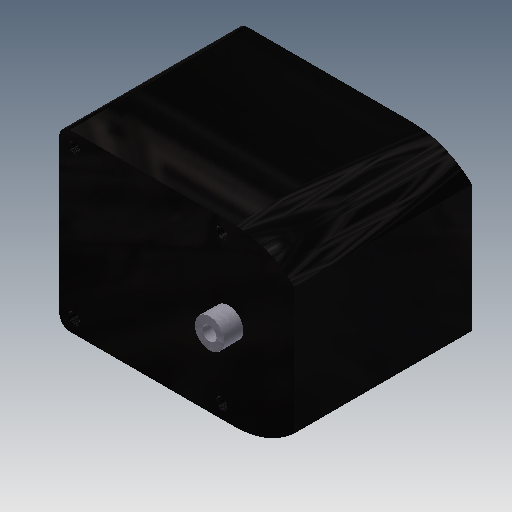
# Autodesk Inventor part: KRS-4034HV
Saved by Autodesk Inventor 2019.4 (Build 234330000, 330)
## iProperties
Created: 2017-04-05
Part Number: KRS-4034HV
Material: アセタール樹脂、黒
Document SubType Name: Modeling
Designer: Owner
Density: 1.41547 g/cm^3
Appearance: 滑らか - 黒
Mass: 61.2 g
Surface Area: 86.4058 cm^2
Volume: 43.2365 cm^3
Author: Owner
Autodesk Inventor part; units mm, degrees
ref_plane "YZ Plane" through (0, 0, 0) normal (1, 0, 0) x (0, 1, 0)
ref_plane "XZ Plane" through (0, 0, 0) normal (0, 1, 0) x (-1, 0, 0)
ref_plane "XY Plane" through (0, 0, 0) normal (0, 0, 1) x (1, 0, 0)
sketch "スケッチ1" plane through (0, 0, 0) normal (0, 0, 1) x (1, 0, 0)
  line L0 (-37.5496, 23.6801) -> (-7.5496, 23.6801)
  line L1 (3.4504, 19.2991) -> (3.4504, -3.9388)
  line L2 (-7.5496, -8.3199) -> (-37.5496, -8.3199)
  line L3 (-39.5496, -6.3199) -> (-39.5496, 21.6801)
  circle A0 centre (-36.8093, -5.8199) radius 1.05
  circle A1 centre (-36.8093, 21.1801) radius 1.05
  arc A2 (-37.5496, 23.6801) -> (-39.5496, 21.6801) centre (-37.5496, 21.6801) ccw
  arc A3 (-39.5496, -6.3199) -> (-37.5496, -8.3199) centre (-37.5496, -6.3199) ccw
  circle A4 centre (-9.8093, -5.8199) radius 1.05
  circle A5 centre (-9.8093, 21.1801) radius 1.05
  line L4 (-39.5496, 7.6801) -> (3.4504, 7.6801) construction
  line L5 (-17.0496, 23.6801) -> (-17.0496, -8.3199) construction
  arc A6 (-7.5496, -8.3199) -> (3.4504, -3.9388) centre (-7.5496, 7.6801) ccw
  arc A7 (3.4504, 19.2991) -> (-7.5496, 23.6801) centre (-7.5496, 7.6801) ccw
  point P0 (-39.5496, -8.3199)
  point P1 (-17.0496, 7.6801)
  dimension "d23" = 2.1
  dimension "d24" = 2.1
  dimension "d25" = 27
  dimension "d26" = 2.5
  dimension "d27" = 2.5
  dimension "d28" = 2
  dimension "d31" = 2.1
  dimension "d32" = 2.1
  dimension "d33" = 27
  dimension "d34" = 27
  constraints: 12 end point, 8 centre point, 8 point on circle, 4 point on line, 4 tangent, 3 midpoint, 2 parallel, 1 equal radius, 1 horizontal, 1 perpendicular
  measures "d23" diameter of A0
  measures "d24" diameter of A1
  measures "d25" distance of A0.centre A1.centre
  measures "d26" distance from line of L0 A1.centre
  measures "d27" distance from line of L2 A0.centre
  measures "d28" radius of A2
  measures "d31" diameter of A4
  measures "d32" diameter of A5
  measures "d33" distance of A0.centre A4.centre
  measures "d34" distance of A5.centre A1.centre
extrude "押し出し1" add sketch "スケッチ1" along normal blind 32.5
sketch "スケッチ2" plane through (0, 0, 32.5) normal (0, 0, 1) x (1, 0, 0)
  circle A0 centre (-9.8093, 21.1801) radius 1.05 projected
  circle A1 centre (-9.8093, -5.8199) radius 1.05 projected
  circle A2 centre (-36.8093, 21.1801) radius 1.05 projected
  circle A3 centre (-36.8093, -5.8199) radius 1.05 projected
  line L0 (3.4504, -3.9388) -> (3.4504, 19.2991) projected
  arc A4 (3.4504, 19.2991) -> (-7.5496, 23.6801) centre (-7.5496, 7.6801) ccw projected
  line L1 (-7.5496, 23.6801) -> (-37.5496, 23.6801) projected
  arc A5 (-37.5496, 23.6801) -> (-39.5496, 21.6801) centre (-37.5496, 21.6801) ccw projected
  line L2 (-39.5496, 21.6801) -> (-39.5496, -6.3199) projected
  arc A6 (-39.5496, -6.3199) -> (-37.5496, -8.3199) centre (-37.5496, -6.3199) ccw projected
  line L3 (-37.5496, -8.3199) -> (-7.5496, -8.3199) projected
  arc A7 (-7.5496, -8.3199) -> (3.4504, -3.9388) centre (-7.5496, 7.6801) ccw projected
  line L4 (-39.5496, 21.6801) -> (-39.5496, -6.3199) construction
  line L5 (-39.5496, 7.6801) -> (3.4504, 7.6801) construction
  line L6 (-7.5496, -8.3199) -> (-37.5496, -8.3199) construction
  line L7 (-18.0496, -8.3199) -> (-18.0496, 23.6801) construction
  line L8 (-7.5496, 23.6801) -> (-37.5496, 23.6801) construction
  circle A8 centre (-8.55, 7.6801) radius 2.7
  circle A9 centre (-8.55, 7.6801) radius 1.3
  point P0 (0, 0)
  dimension "d49" = 5.4
  dimension "d50" = 2.6
  dimension "d51" = 9.4996
  constraints: 4 end point, 3 point on line, 2 centre point, 2 coincident, 2 midpoint, 1 perpendicular
  measures "d49" diameter of A8
  measures "d50" diameter of A9
  measures "d51" distance from line of L7 A8.centre
extrude "押し出し3" add sketch "スケッチ2" along normal blind 3.5 contours A8
sketch "スケッチ3" plane through (0, 0, 0) normal (0, 0, -1) x (-1, 0, 0)
  circle A0 centre (9.8093, 21.1801) radius 1.05 projected
  circle A1 centre (9.8093, -5.8199) radius 1.05 projected
  circle A2 centre (36.8093, 21.1801) radius 1.05 projected
  circle A3 centre (36.8093, -5.8199) radius 1.05 projected
  line L0 (-3.4504, 19.2991) -> (-3.4504, -3.9388) projected
  arc A4 (-3.4504, -3.9388) -> (7.5496, -8.3199) centre (7.5496, 7.6801) ccw projected
  line L1 (7.5496, -8.3199) -> (37.5496, -8.3199) projected
  arc A5 (37.5496, -8.3199) -> (39.5496, -6.3199) centre (37.5496, -6.3199) ccw projected
  line L2 (39.5496, -6.3199) -> (39.5496, 21.6801) projected
  arc A6 (39.5496, 21.6801) -> (37.5496, 23.6801) centre (37.5496, 21.6801) ccw projected
  line L3 (37.5496, 23.6801) -> (7.5496, 23.6801) projected
  arc A7 (7.5496, 23.6801) -> (-3.4504, 19.2991) centre (7.5496, 7.6801) ccw projected
  line L4 (39.5496, -6.3199) -> (39.5496, 21.6801) construction
  line L5 (39.5496, 7.6801) -> (-3.4504, 7.6801) construction
  line L6 (-3.4504, 19.2991) -> (-3.4504, -3.9388) construction
  line L7 (7.5496, -8.3199) -> (37.5496, -8.3199) construction
  line L8 (18.0496, -8.3199) -> (18.0496, 23.6801) construction
  line L9 (37.5496, 23.6801) -> (7.5496, 23.6801) construction
  circle A8 centre (8.55, 7.6801) radius 1.3
  circle A9 centre (31.5496, -5.8199) radius 1.05
  circle A10 centre (18.5496, 21.1801) radius 1.05
  circle A11 centre (1.0496, 18.3126) radius 1.05
  circle A12 centre (1.0496, -3.6874) radius 1.05
  point P0 (0, 0)
  dimension "d54" = 2.6
  dimension "d55" = 2.1
  dimension "d56" = 13.5
  dimension "d57" = 2.1
  dimension "d58" = 0.5
  dimension "d59" = 2.1
  dimension "d60" = 17
  dimension "d61" = 2.1
  dimension "d62" = 22
  dimension "d63" = 17
  constraints: 5 centre point, 4 end point, 3 point on line, 2 midpoint, 1 coincident, 1 perpendicular
  measures "d54" diameter of A8
  measures "d55" diameter of A9
  measures "d56" distance from line of A9.centre L8
  measures "d57" diameter of A10
  measures "d58" distance from line of L8 A10.centre
  measures "d59" diameter of A11
  measures "d60" distance from line of L8 A11.centre
  measures "d61" diameter of A12
  measures "d62" distance of A11.centre A12.centre
  measures "d63" distance from line of L8 A12.centre
extrude "押し出し4" cut sketch "スケッチ3" against normal blind 10 contours A8 | A9 | A10 | A11 | A12
sketch "スケッチ4" plane through (-37.5496, -8.3199, 0) normal (0, -1, 0) x (1, 0, 0)
  line L0 (30, 0) -> (0, 0) projected
  line L1 (30, 0) -> (30, 32.5) projected
  line L2 (0, 32.5) -> (30, 32.5) projected
  line L3 (0, 0) -> (0, 32.5) projected
  line L4 (0, 0) -> (-2, 0) projected
  line L5 (0, 0) -> (0, 32.5) projected
  line L6 (-2, 32.5) -> (0, 32.5) projected
  line L7 (-2, 0) -> (-2, 32.5) projected
  line L8 (41, 0) -> (30, 0) projected
  line L9 (41, 0) -> (41, 32.5) projected
  line L10 (30, 32.5) -> (41, 32.5) projected
  line L11 (30, 0) -> (30, 32.5) projected
  line L12 (0, 32.5) -> (30, 32.5) construction
  line L13 (19.5, 32.5) -> (19.5, 0) construction
  line L14 (17.5, 10.5) -> (25.5, 10.5)
  line L15 (25.5, 10.5) -> (25.5, 5)
  line L16 (25.5, 5) -> (17.5, 5)
  line L17 (17.5, 5) -> (17.5, 10.5)
  point P0 (37.5496, 0)
  dimension "d66" = 21.5
  dimension "d67" = 8
  dimension "d68" = 5.5
  dimension "d69" = 5
  dimension "d70" = 2
  constraints: 10 end point, 2 parallel, 2 perpendicular, 2 point on line, 1 horizontal
  measures "d66" distance between parallel lines of L13 L7
  measures "d67" distance of L15.end L16.end
  measures "d68" distance of L14.end L15.end
  measures "d69" distance between parallel lines of L0 L16
  measures "d70" distance between parallel lines of L13 L17
extrude "押し出し5" add sketch "スケッチ4" along normal blind 3 contours L14 L15 L16 L17
